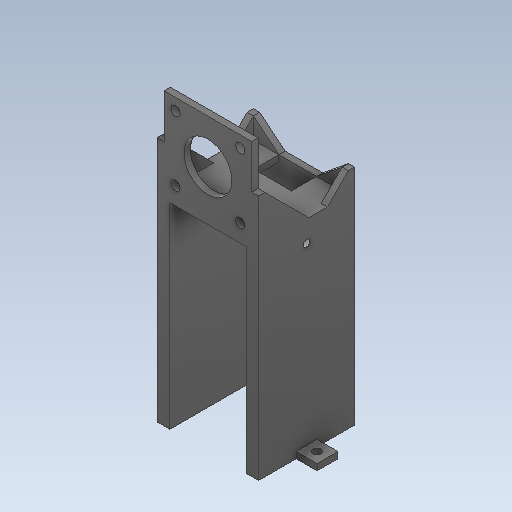
# Autodesk Inventor part: Torre Motor Definitiva Pont
Saved by Autodesk Inventor 2021 (Build 250183000, 183)
## iProperties
Created: 2021-04-07
Part Number: Torre Motor Definitiva Pont
Material: Plástico ABS
Document SubType Name: Modeling
Designer: Marc
Density: 1.06 g/cm^3
Appearance: Suave - Blanco
Author: Marc
Autodesk Inventor part; units mm, degrees
ref_plane "YZ Plane" through (0, 0, 0) normal (1, 0, 0) x (0, 1, 0)
ref_plane "XZ Plane" through (0, 0, 0) normal (0, 1, 0) x (-1, 0, 0)
ref_plane "XY Plane" through (0, 0, 0) normal (0, 0, 1) x (1, 0, 0)
sketch "Boceto1" plane through (0, 0, 0) normal (0, 0, 1) x (1, 0, 0)
  line L0 (-21, 21) -> (21, 21)
  line L1 (21, 21) -> (21, -21)
  line L2 (21, -21) -> (-21, -21)
  line L3 (-21, -21) -> (-21, 21)
  circle A0 centre (0, 0) radius 11.5
  circle A1 centre (-15.5, 15.5) radius 2.25
  circle A2 centre (-15.5, -15.5) radius 2.25
  circle A3 centre (15.5, -15.5) radius 2.25
  circle A4 centre (15.5, 15.5) radius 2.25
  dimension "d0" = 42
  dimension "d1" = 42
  dimension "d2" = 23
  dimension "d6" = 4.5
  dimension "d7" = 4.5
  dimension "d8" = 4.5
  dimension "d9" = 4.5
  constraints: 8 end point, 5 centre point, 2 parallel, 1 coincident, 1 horizontal, 1 perpendicular
  measures "d0" distance of L1.end L2.end
  measures "d1" distance of L0.end L1.end
  measures "d2" diameter of A0
  measures "d6" diameter of A1
  measures "d7" diameter of A2
  measures "d8" diameter of A3
  measures "d9" diameter of A4
extrude "Extrusión1" add sketch "Boceto1" along normal blind 3
sketch "Boceto28" plane through (0, 0, 3) normal (0, 0, 1) x (1, 0, 0)
  line L0 (-21.25, -24) -> (21.25, -24)
  line L1 (21.25, -24) -> (21.25, -21)
  line L2 (-21.25, -21) -> (-21.25, -24)
  line L3 (-21, -21) -> (21, -21) projected
  line L4 (21.25, -21) -> (-21.25, -21)
  point P0 (0, 0)
  constraints: 8 end point, 1 horizontal, 1 parallel, 1 perpendicular
extrude "Extrusión24" add sketch "Boceto28" against normal blind 43
sketch "Boceto29" plane through (-21.25, -21, -40) normal (0, 1, 0) x (1, 0, 0)
  line L0 (30.25, -12) -> (12.25, -12)
  line L1 (0, 0) -> (42.5, 0) projected
  line L2 (12.25, 0) -> (30.25, 0)
  line L3 (12.25, 0) -> (12.25, -12)
  line L4 (30.25, 0) -> (30.25, -12)
  point P0 (21.25, -40)
  constraints: 8 end point, 2 point on line, 1 parallel, 1 vertical
extrude "Extrusión25" cut sketch "Boceto29" against normal blind 3
sketch "Boceto33" plane through (21.25, -24, 3) normal (1, 0, 0) x (0, 0, -1)
  line L0 (43, 0) -> (33, 0)
  line L1 (33, 0) -> (33, 3)
  line L2 (43, 0) -> (46, 0)
  line L3 (46, 0) -> (46, 13)
  line L4 (46, 13) -> (43, 13)
  line L5 (43, 13) -> (33, 3)
  line L6 (0, 45) -> (0, 3) projected
  line L7 (0, 0) -> (43, 0) projected
  line L8 (0, 24) -> (0, 0)
  line L9 (0, 0) -> (24, 0)
  line L10 (24, 0) -> (24, 3)
  line L11 (0, 3) -> (43, 3) projected
  line L12 (0, 24) -> (3, 24)
  line L13 (3, 45) -> (3, 3) projected
  line L14 (3, 24) -> (24, 3)
  point P0 (0, 3)
  dimension "d153" = 10
  dimension "d154" = 3
  dimension "d155" = 13
  dimension "d156" = 3
  dimension "d181" = 24
  constraints: 22 end point, 5 perpendicular, 2 midpoint, 1 horizontal, 1 point on line
  measures "d153" distance of L0.start L0.end
  measures "d154" distance of L0.start L2.end
  measures "d155" distance of L2.end L3.end
  measures "d156" distance of L3.end L4.end
  measures "d181" distance of L7.start L9.end
extrude "Extrusión28" add sketch "Boceto33" along normal blind 3 contours L0 L1 L5 L4 L3 L2 | L7 L8 L11 L10 | L11 L13 L14 | L11 L6 L12 L13
sketch "Boceto34" plane through (-21.25, -24, 3) normal (-1, 0, 0) x (0, 0, 1)
  line L0 (-46, 0) -> (-46, 13) projected
  line L1 (-46, 13) -> (-43, 13) projected
  line L2 (-46, 13) -> (-43, 13)
  line L3 (-43, 13) -> (-33, 3)
  line L4 (-43, 0) -> (-46, 0) projected
  line L5 (-46, 13) -> (-46, 0)
  line L6 (-46, 0) -> (-33, 0)
  line L7 (-33, 3) -> (-33, 0)
  line L8 (-24, 0) -> (-24, 3)
  line L9 (-24, 3) -> (-3, 24)
  line L10 (0, 24) -> (-3, 24)
  line L11 (-24, 0) -> (0, 0)
  line L12 (0, 0) -> (0, 24)
  constraints: 20 end point, 3 perpendicular, 1 horizontal, 1 vertical
extrude "Extrusión29" add sketch "Boceto34" along normal blind 3
sketch "Boceto36" plane through (0, 0, -40) normal (0, 0, -1) x (-1, 0, 0)
  line L0 (9, -21) -> (9, -24) projected
  line L1 (9, -24) -> (21.25, -24)
  line L2 (21.25, -24) -> (21.25, -11)
  line L3 (9, -21) -> (9, -24)
  line L4 (-9, -24) -> (-9, -21) projected
  line L5 (-9, -21) -> (-9, -24)
  line L6 (-21, -21) -> (-21, 21) projected
  line L7 (-21.25, -11) -> (-9, -21)
  line L8 (-21.25, -11) -> (-21.25, -24)
  line L9 (24.25, -24) -> (-24.25, -24) projected
  line L10 (-9, -24) -> (-21.25, -24)
  line L11 (9, -21) -> (21.25, -11)
  constraints: 16 end point, 2 perpendicular, 1 horizontal, 1 parallel, 1 point on line, 1 vertical
extrude "Extrusión31" add sketch "Boceto36" along normal blind 3
sketch "Boceto37" plane through (-21, -21, 0) normal (0, 1, 0) x (1, 0, 0)
  line L0 (45.25, 40) -> (45.25, 30) projected
  line L1 (42.25, 21) -> (42.25, 0) projected
  line L2 (45.25, 30) -> (42.25, 30)
  line L3 (42.25, 30) -> (42.25, 21)
  line L4 (42.25, 21) -> (45.25, 21)
  line L5 (45.25, 21) -> (45.25, 30)
  line L6 (30, 40) -> (30, 43) projected
  line L7 (12, 43) -> (12, 28) projected
  line L8 (30, 40) -> (12, 40)
  line L9 (12, 40) -> (12, 43)
  line L10 (12, 43) -> (30, 43)
  line L11 (30, 43) -> (30, 40)
  line L12 (-0.25, 21) -> (-0.25, 30) projected
  line L13 (-3.25, 0) -> (-3.25, 21) projected
  line L14 (-0.25, 30) -> (-3.25, 30)
  line L15 (-3.25, 30) -> (-3.25, 21)
  line L16 (-3.25, 21) -> (-0.25, 21)
  line L17 (-0.25, 21) -> (-0.25, 30)
  constraints: 24 end point, 6 parallel, 3 horizontal, 3 perpendicular
extrude "Extrusión32" add sketch "Boceto37" against normal blind 3
sketch "Boceto38" plane through (0, 0, 3) normal (0, 0, 1) x (1, 0, 0)
  line L0 (-21.25, 0) -> (-21.25, -21) projected
  line L1 (-21, -21) -> (-21.25, -21) projected
  line L2 (-21.25, 0) -> (-21, 0)
  line L3 (-21, 0) -> (-21, -21)
  line L4 (-21, -21) -> (-21.25, -21)
  line L5 (-21.25, -21) -> (-21.25, 0)
  line L6 (21, -21) -> (21, 21) projected
  line L7 (21.25, 0) -> (21.25, -21) projected
  line L8 (21, -21) -> (21.25, -21)
  line L9 (21.25, -21) -> (21.25, 0)
  line L10 (21.25, 0) -> (21, 0)
  line L11 (21, 0) -> (21, -21)
  constraints: 16 end point, 4 parallel, 2 horizontal, 2 perpendicular
extrude "Extrusión33" add sketch "Boceto38" against normal blind 3
sketch "Boceto50" plane through (24.25, -24, -43) normal (0, -1, 0) x (1, 0, 0)
  line L0 (-45.5, 0) -> (-48.5, 0) projected
  line L1 (-48.5, 0) -> (-48.5, 46) projected
  line L2 (-48.5, 0) -> (-48.5, 46)
  line L3 (-48.5, 46) -> (-42.5, 46)
  line L4 (-42.5, 46) -> (-42.5, 3)
  line L5 (-48.5, 0) -> (0, 0) projected
  line L6 (-48.5, 0) -> (0, 0)
  line L7 (0, 0) -> (0, 46)
  line L8 (0, 46) -> (-6, 46)
  line L9 (-6, 46) -> (-6, 3)
  line L10 (-42.5, 3) -> (-6, 3)
  dimension "d183" = 6
  dimension "d184" = 6
  constraints: 16 end point, 5 perpendicular, 2 collinear
  measures "d183" distance of L1.end L3.end
  measures "d184" distance of L7.end L8.end
extrude "Extrusión39" add sketch "Boceto50" along normal blind 94
sketch "Boceto51" plane through (24.25, -24, 3) normal (1, 0, 0) x (0, 0, -1)
  line L0 (18, -94) -> (28, -94)
  line L1 (28, -94) -> (28, -91)
  line L2 (28, -91) -> (18, -91)
  line L3 (18, -91) -> (18, -94)
  point P0 (3, 24)
  dimension "d171" = 10
  dimension "d172" = 3
  constraints: 8 end point, 2 parallel, 1 horizontal, 1 perpendicular
  measures "d171" distance of L2.end L1.end
  measures "d172" distance of L1.end L0.end
extrude "Extrusión40" add sketch "Boceto51" along normal blind 10
sketch "Boceto52" plane through (-24.25, -24, 3) normal (-1, 0, 0) x (0, 0, 1)
  line L0 (0, -94) -> (-46, -94) projected
  line L1 (-18, -91) -> (-18, -94) projected
  line L2 (-23, -94) -> (-18, -94)
  line L3 (-18, -94) -> (-18, -91)
  line L4 (-28, -91) -> (-18, -91) projected
  line L5 (-18, -91) -> (-28, -91)
  line L6 (-28, -94) -> (-28, -91) projected
  line L7 (-28, -91) -> (-28, -94)
  line L8 (-28, -94) -> (-23, -94)
  point P0 (-3, 24)
  constraints: 10 end point, 3 perpendicular, 2 collinear, 1 midpoint
extrude "Extrusión41" add sketch "Boceto52" along normal blind 10
sketch "Boceto56" plane through (-24.25, -115, -15) normal (0, 1, 0) x (1, 0, 0)
  line L0 (48.5, 0) -> (58.5, 0) projected
  line L1 (48.5, 10) -> (58.5, 10) projected
  line L2 (0, 10) -> (-10, 10) projected
  line L3 (0, 0) -> (-10, 0) projected
  line L4 (-10, 0) -> (-10, 10) projected
  circle A0 centre (-5, 5) radius 2
  circle A1 centre (53.5, 5) radius 2
  point P0 (24.25, -15)
  dimension "d185" = 4
  dimension "d186" = 4
  constraints: 2 centre point
  measures "d185" diameter of A0
  measures "d186" diameter of A1
extrude "Extrusión43" cut sketch "Boceto56" against normal blind 3
sketch "Boceto66" plane through (24.25, -24, 3) normal (1, 0, 0) x (0, 0, -1)
  line L0 (3, 24) -> (24, 3) projected
  circle A0 centre (23, -7) radius 1.6
  dimension "d224" = 3.2
  constraints: 1 centre point
  measures "d224" diameter of A0
extrude "Extrusión48" cut sketch "Boceto66" against normal blind 10
sketch "Boceto67" plane through (-24.25, -24, 3) normal (-1, 0, 0) x (0, 0, 1)
  line L0 (0, 24) -> (0, -94) projected
  circle A0 centre (-23, -7) radius 1.6
  point P0 (-3, 24)
  point P1 (-24, 3)
  dimension "d228" = 3.2
  constraints: 1 centre point
  measures "d228" diameter of A0
extrude "Extrusión50" cut sketch "Boceto67" against normal blind 10
